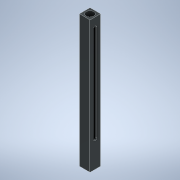
# Autodesk Inventor part: telescopic boom1
Saved by Autodesk Inventor 2021 (Build 250183000, 183)
## iProperties
Created: 2020-12-24
Part Number: telescopic boom1
Material: PVC-Piping
Document SubType Name: Modeling
Designer: Vikki
Density: 1.4 g/cm^3
Appearance: Iron Gray
Mass: 72.921 g
Surface Area: 299.002 cm^2
Volume: 52.0864 cm^3
Author: Vikki
Autodesk Inventor part; units mm, degrees
ref_plane "XZ Plane" through (0, 0, 0) normal (0, 1, 0) x (-1, 0, 0)
ref_plane "XY Plane" through (0, 0, 0) normal (0, 0, 1) x (1, 0, 0)
sketch "Sketch1" plane through (0, 0, 0) normal (0, 1, 0) x (-1, 0, 0)
  circle A0 centre (0, 0) radius 7.25
  circle A1 centre (0, 0) radius 4.75 construction
  circle A2 centre (0, 0) radius 10
  dimension "d0" = 14.5
  dimension "d1" = 2.5
  dimension "d4" = 20
  constraints: 3 centre point, 3 coincident
  measures "d0" diameter of A0
  measures "d1" radial gap between concentric circles of A0 A1
  measures "d4" diameter of A2
extrude "Extrusion1" add sketch "Sketch1" along normal blind 250
ref_plane "Work Plane1" through (10, 0, 0) normal (1, 0, 0) x (0, 1, 0)
sketch "Sketch2" plane through (10, 0, 0) normal (1, 0, 0) x (0, 1, 0)
  line L0 (50, 0) -> (232, 0) construction
  line L1 (50, 3) -> (232, 3)
  line L2 (232, -3) -> (50, -3)
  arc A0 (50, 3) -> (50, -3) centre (50, 0) ccw
  arc A1 (232, -3) -> (232, 3) centre (232, 0) ccw
  line L3 (250, -10) -> (250, 10) projected
  point P0 (0, 0)
  point P1 (141, 0)
  dimension "d6" = 50
  dimension "d7" = 3
  dimension "d10" = 18
  constraints: 8 end point, 4 point on circle, 4 tangent, 2 centre point, 1 horizontal, 1 horizontal alignment, 1 midpoint, 1 parallel
  measures "d6" distance of point (0, 0) L0.start
  measures "d7" radius of A1
  measures "d10" distance from line of L3 L0.end
extrude "Extrusion2" cut sketch "Sketch2" against normal through all
sketch "Sketch3" plane through (0, 0, 0) normal (0, -1, 0) x (1, 0, 0)
  line L0 (10, -10) -> (-10, -10)
  line L1 (-10, -10) -> (-10, 10)
  line L2 (-10, 10) -> (10, 10)
  line L3 (10, 10) -> (10, -10)
  line L4 (10, -10) -> (-10, 10) construction
  line L5 (-10, -10) -> (10, 10) construction
  circle A0 centre (0, 0) radius 10 projected
  point P0 (-10, 0)
  point P1 (0, 10)
  point P2 (10, 0)
  point P3 (0, -10)
  constraints: 12 end point, 2 midpoint, 2 parallel, 2 tangent, 1 horizontal, 1 perpendicular
extrude "Extrusion3" add sketch "Sketch3" against normal up to surface (250 mm away) contours L0 A0 L3 | L0 L1 A0 | A0 L2 L3 | L1 L2 A0
sketch "Sketch4" plane through (10, 0, 10) normal (1, 0, 0) x (0, 0, -1)
  line L0 (13, 50) -> (13, 232) projected
  spline S0 degree 5 poles (13, 232) (13, 232.4388) (12.9195, 232.8782) (12.7598, 233.3002) (12.5191, 233.6988) (12.0539, 234.1957) (11.9027, 234.3331) (11.7356, 234.461) (11.5521, 234.577) (11.1181, 234.7963) (10.8621, 234.8935) (10.583, 234.9646) (10.2918, 235) (9.7112, 235) (9.4219, 234.9651) (9.1472, 234.8959) (8.8921, 234.8001) (8.4576, 234.583) (8.2724, 234.4668) (8.1037, 234.3385) (7.9512, 234.2006) (7.4832, 233.7026) (7.2413, 233.3032) (7.0809, 232.8803) (7, 232.4398) (7, 232) knots 0 0 0 0 0 0 0.263254 0.263254 0.263254 0.263254 0.37209 0.37209 0.37209 0.37209 0.500061 0.500061 0.500061 0.500061 0.626701 0.626701 0.626701 0.626701 0.736162 0.736162 0.736162 0.736162 1 1 1 1 1 1 projected
  line L1 (7, 232) -> (7, 50) projected
  spline S1 degree 5 poles (7, 50) (7, 49.5612) (7.0805, 49.1218) (7.2402, 48.6998) (7.4809, 48.3012) (7.9461, 47.8043) (8.0973, 47.6669) (8.2644, 47.539) (8.4479, 47.423) (8.8819, 47.2037) (9.1379, 47.1065) (9.417, 47.0354) (9.7082, 47) (10.2888, 47) (10.5781, 47.0349) (10.8528, 47.1041) (11.1079, 47.1999) (11.5424, 47.417) (11.7276, 47.5332) (11.8963, 47.6615) (12.0488, 47.7994) (12.5168, 48.2974) (12.7587, 48.6968) (12.9191, 49.1197) (13, 49.5602) (13, 50) knots 0 0 0 0 0 0 0.263254 0.263254 0.263254 0.263254 0.37209 0.37209 0.37209 0.37209 0.500061 0.500061 0.500061 0.500061 0.626701 0.626701 0.626701 0.626701 0.736162 0.736162 0.736162 0.736162 1 1 1 1 1 1 projected
  point P0 (10, 0)
  constraints: 2 horizontal alignment
extrude "Extrusion4" cut sketch "Sketch4" against normal up to surface (20 mm away)
body "Solid1"
